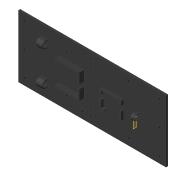
# Autodesk Inventor part: lowerBase
Saved by Autodesk Inventor 2019 (Build 230136000, 136)
## iProperties
Created: 2021-03-03
Part Number: lowerBase
Material: Generic
Document SubType Name: Modeling
Designer: LuoYi
Density: 1 g/cm^3
Appearance: Default
Author: LuoYi
Autodesk Inventor part; units mm, degrees
ref_plane "YZ Plane" through (0, 0, 0) normal (1, 0, 0) x (0, 1, 0)
ref_plane "XZ Plane" through (0, 0, 0) normal (0, 1, 0) x (-1, 0, 0)
ref_plane "XY Plane" through (0, 0, 0) normal (0, 0, 1) x (1, 0, 0)
sketch "Sketch1" plane through (0, 0, 0) normal (0, 0, 1) x (1, 0, 0)
  line L0 (0, 0) -> (200, 0)
  line L1 (200, 0) -> (200, 100)
  line L2 (200, 100) -> (0, 100)
  line L3 (0, 100) -> (0, 0)
  dimension "d0" = 200
  dimension "d1" = 100
  constraints: 8 end point, 2 parallel, 1 horizontal, 1 perpendicular
  measures "d0" distance of L2.end L1.end
  measures "d1" distance of L1.end L0.end
extrude "Extrusion1" add sketch "Sketch1" along normal blind 3
sketch "Sketch2" plane through (0, 0, 2) normal (-1, 0, 0) x (0, 0, 1)
  line L0 (1, 0) -> (1, 100) projected
  line L1 (1, 81.5) -> (5, 81.5)
  arc A0 (5, 73.5) -> (5, 81.5) centre (5, 77.5) ccw
  line L2 (5, 73.5) -> (1, 73.5)
  arc A1 (5, 71.5) -> (5, 83.5) centre (5, 77.5) ccw
  line L3 (5, 83.5) -> (1, 83.5)
  line L4 (5, 71.5) -> (1, 71.5)
  line L5 (1, 28.5) -> (5, 28.5)
  arc A2 (5, 16.5) -> (5, 28.5) centre (5, 22.5) ccw
  line L6 (5, 16.5) -> (1, 16.5)
  line L7 (1, 26.5) -> (5, 26.5)
  arc A3 (5, 18.5) -> (5, 26.5) centre (5, 22.5) ccw
  line L8 (5, 18.5) -> (1, 18.5)
  line L9 (1, 50) -> (8.8605, 50) construction
  line L10 (5, 77.5) -> (5, 22.5) construction
  point P0 (-2, 0)
  point P1 (5, 50)
  dimension "d4" = 8
  dimension "d5" = 2
  dimension "d6" = 2
  dimension "d7" = 8
  dimension "d8" = 55
  dimension "d9" = 4
  constraints: 20 end point, 9 horizontal, 8 point on circle, 8 tangent, 4 centre point, 2 coincident, 1 midpoint, 1 point on line, 1 vertical, 10 other
  measures "d4" distance between parallel lines of L8 L7
  measures "d5" distance between parallel lines of L5 L7
  measures "d6" distance between parallel lines of L2 L4
  measures "d7" distance between parallel lines of L2 L1
  measures "d8" distance of L10.start L10.end
extrude "Extrusion2" add sketch "Sketch2" against normal blind 10 contours L0 L2 A0 L1 L3 A1 L4 | L0 L8 A3 L7 L5 A2 L6
sketch "Sketch3" plane through (0, 0, 3) normal (0, 0, 1) x (1, 0, 0)
  line L0 (0, 71.5) -> (0, 28.5) projected
  line L1 (0, 50) -> (200, 50) construction
  line L2 (200, 0) -> (200, 100) projected
  line L3 (68, 30) -> (28, 30)
  line L4 (28, 30) -> (28, 70)
  line L5 (28, 70) -> (68, 70)
  line L6 (68, 70) -> (68, 30)
  line L7 (68, 30) -> (28, 70) construction
  line L8 (28, 30) -> (68, 70) construction
  line L9 (66, 32) -> (30, 32)
  line L10 (30, 32) -> (30, 68)
  line L11 (30, 68) -> (66, 68)
  line L12 (66, 68) -> (66, 32)
  line L13 (66, 32) -> (30, 68) construction
  line L14 (30, 32) -> (66, 68) construction
  line L15 (30, 68) -> (28, 68)
  line L16 (28, 68) -> (28, 32)
  line L17 (28, 32) -> (30, 32)
  line L18 (30, 32) -> (30, 68)
  line L19 (66, 46.75) -> (68, 46.75)
  line L20 (68, 46.75) -> (68, 53.25)
  line L21 (68, 53.25) -> (66, 53.25)
  line L22 (66, 53.25) -> (66, 46.75)
  point P0 (0, 0)
  point P1 (48, 50)
  point P2 (48, 50)
  point P3 (66, 50)
  dimension "d15" = 36
  dimension "d17" = 36
  dimension "d18" = 2
  dimension "d19" = 2
  dimension "d20" = 28
  dimension "d23" = 6.5
  constraints: 42 end point, 9 midpoint, 8 parallel, 4 horizontal, 4 perpendicular, 4 point on line, 1 collinear
  measures "d15" distance between parallel lines of L12 L10
  measures "d17" distance of L9.end L10.end
  measures "d18" distance between parallel lines of L5 L11
  measures "d19" distance between parallel lines of L4 L10
  measures "d20" distance between parallel lines of L0 L4
  measures "d23" distance between parallel lines of L21 L19
extrude "Extrusion3" add sketch "Sketch3" along normal blind 8 contours L3 L4 L17 L9 L12 L19 L6 | L21 L12 L11 L15 L4 L5 L6
sketch "Sketch4" plane through (0, 0, 3) normal (0, 0, 1) x (1, 0, 0)
  line L0 (0, 71.5) -> (0, 28.5) projected
  line L1 (200, 0) -> (200, 100) projected
  line L2 (100, 59) -> (130.2, 59)
  line L3 (130.2, 59) -> (130.2, 34.5)
  line L4 (130.2, 34.5) -> (100, 34.5)
  line L5 (100, 34.5) -> (100, 59)
  line L6 (98, 61) -> (132.2, 61)
  line L7 (132.2, 61) -> (132.2, 32.5)
  line L8 (132.2, 32.5) -> (98, 32.5)
  line L9 (98, 32.5) -> (98, 61)
  line L10 (88, 53.6) -> (98, 53.6) construction
  line L11 (98, 46.4) -> (88, 46.4) construction
  line L12 (88, 46.4) -> (88, 53.6) construction
  line L13 (88, 50) -> (0, 50) construction
  line L14 (68, 53.25) -> (68, 70) projected
  line L15 (98, 53.6) -> (100, 53.6)
  line L16 (98, 46.4) -> (100, 46.4)
  line L17 (130.2, 53.6) -> (132.2, 53.6)
  line L18 (130.2, 46.4) -> (132.2, 46.4)
  line L19 (105.149, 34.5) -> (105.149, 32.5)
  line L20 (129.3871, 34.5) -> (129.3871, 32.5)
  point P0 (0, 0)
  dimension "d24" = 24.5
  dimension "d25" = 30.2
  dimension "d26" = 2
  dimension "d27" = 2
  dimension "d28" = 2
  dimension "d29" = 2
  dimension "d30" = 7.2
  dimension "d31" = 10
  dimension "d32" = 20
  dimension "d33" = 9
  constraints: 36 end point, 16 point on line, 6 perpendicular, 5 parallel, 4 horizontal, 2 midpoint
  measures "d24" distance between parallel lines of L4 L2
  measures "d25" distance between parallel lines of L3 L5
  measures "d26" distance between parallel lines of L9 L5
  measures "d27" distance between parallel lines of L6 L2
  measures "d28" distance between parallel lines of L7 L3
  measures "d29" distance between parallel lines of L8 L4
  measures "d30" distance between parallel lines of L11 L10
  measures "d31" distance of L11.start L11.end
  measures "d32" distance between parallel lines of L14 L12
  measures "d33" distance between parallel lines of L2 L13
extrude "Extrusion4" add sketch "Sketch4" along normal blind 5 contours L5 L15 L9 L6 L7 L17 L3 L2 | L5 L4 L19 L8 L9 L16 | L18 L7 L8 L20 L4 L3
sketch "Sketch5" plane through (0, 0, 0) normal (-1, 0, 0) x (0, 0, 1)
  line L0 (0, 0) -> (0, 100) projected
  line L1 (3, 0) -> (3, 100) projected
  line L2 (0, 0) -> (3, 0)
  line L3 (3, 0) -> (3, 100)
  line L4 (3, 100) -> (0, 100)
  line L5 (0, 100) -> (0, 0)
  constraints: 8 end point, 2 parallel, 1 horizontal, 1 perpendicular
extrude "Extrusion5" add sketch "Sketch5" along normal blind 38
sketch "Sketch6" plane through (0, 0, 3) normal (0, 0, 1) x (1, 0, 0)
  circle A0 centre (-28, 10) radius 1.6
  circle A1 centre (140, 10) radius 1.6
  circle A2 centre (190, 10) radius 1.6
  circle A3 centre (190, 50) radius 1.6
  circle A4 centre (190, 90) radius 1.6
  circle A5 centre (140, 90) radius 1.6
  circle A6 centre (-28, 90) radius 1.6
  line L0 (-28, 90) -> (190, 90) construction
  line L1 (190, 90) -> (190, 10) construction
  line L2 (190, 10) -> (-28, 10) construction
  line L3 (-28, 10) -> (-28, 90) construction
  line L4 (200, 100) -> (-38, 100) projected
  line L5 (-38, 0) -> (-38, 100) projected
  line L6 (200, 0) -> (-38, 0) projected
  line L7 (200, 0) -> (200, 100) projected
  line L8 (-38, 50) -> (200, 50) construction
  circle A7 centre (-28, 50) radius 1.6
  line L9 (0, 83.5) -> (0, 71.5) projected
  line L10 (140, 90) -> (140, 10) construction
  line L11 (40, 80) -> (78.5, 80) construction
  line L12 (78.5, 80) -> (78.5, 20) construction
  line L13 (78.5, 20) -> (40, 20) construction
  line L14 (40, 20) -> (40, 80) construction
  circle A8 centre (40, 80) radius 1.6
  circle A9 centre (78.5, 80) radius 1.6
  circle A10 centre (40, 20) radius 1.6
  circle A11 centre (78.5, 20) radius 1.6
  point P0 (0, 0)
  dimension "d38" = 3.2
  dimension "d41" = 3.2
  dimension "d42" = 3.2
  dimension "d43" = 3.2
  dimension "d44" = 3.2
  dimension "d45" = 3.2
  dimension "d48" = 3.2
  dimension "d49" = 10
  dimension "d50" = 10
  dimension "d51" = 10
  dimension "d52" = 10
  dimension "d53" = 3.2
  dimension "d56" = 50
  dimension "d68" = 60
  dimension "d69" = 3.2
  dimension "d70" = 3.2
  dimension "d71" = 3.2
  dimension "d72" = 3.2
  dimension "d73" = 40
  dimension "d74" = 38.5
  constraints: 20 end point, 12 centre point, 4 coincident, 4 midpoint, 4 parallel, 3 point on line, 2 horizontal, 2 perpendicular, 1 vertical, 1 other
  measures "d38" diameter of A0
  measures "d41" diameter of A1
  measures "d42" diameter of A2
  measures "d43" diameter of A3
  measures "d44" diameter of A4
  measures "d45" diameter of A5
  measures "d48" diameter of A6
  measures "d49" distance between parallel lines of L4 L0
  measures "d50" distance between parallel lines of L5 L3
  measures "d51" distance between parallel lines of L6 L2
  measures "d52" distance between parallel lines of L7 L1
  measures "d53" diameter of A7
  measures "d56" distance of L10.start L0.end
  measures "d68" distance of L13.end L11.start
  measures "d69" diameter of A8
  measures "d70" diameter of A9
  measures "d71" diameter of A10
  measures "d72" diameter of A11
  measures "d73" distance between parallel lines of L9 L14
  measures "d74" distance of L11.start L11.end
extrude "Extrusion6" cut sketch "Sketch6" against normal blind 5 contours A0 | A1 | A2 | A3 | A4 | A5 | A6 | A7 | A8 | A9 | A10 | A11
ref_plane "Work Plane1" through (152.2, 32.5, 3) normal (1, 0, 0) x (0, 0, -1)
sketch "Sketch7" plane through (152.2, 32.5, 3) normal (1, 0, 0) x (0, 0, -1)
  line L0 (0, 13.9) -> (0, 2) projected
  line L1 (0, 13) -> (-5, 13)
  arc A0 (-5, 22) -> (-5, 13) centre (-5, 17.5) ccw
  line L2 (-5, 22) -> (0, 22)
  line L3 (0, 21.1) -> (0, 28.5) projected
  arc A1 (-5, 21) -> (-5, 14) centre (-5, 17.5) ccw
  line L4 (-5, 14) -> (0, 14)
  line L5 (-5, 21) -> (0, 21)
  line L6 (0, -32.5) -> (0, 67.5) projected
  line L7 (0, 13.9) -> (-5, 13.9) projected
  line L8 (0, 21.1) -> (-5, 21.1) projected
  line L9 (-5, 13.9) -> (-5, 21.1) construction
  line L10 (-5, 17.5) -> (-5, 17.5) construction
  point P0 (3, -32.5)
  point P1 (0, 0)
  dimension "d63" = 3.5
  dimension "d64" = 4.5
  dimension "d65" = 5
  constraints: 12 end point, 4 horizontal, 4 point on circle, 3 point on line, 2 centre point, 2 perpendicular, 1 coincident, 1 midpoint, 1 tangent, 2 other
  measures "d63" radius of A1
  measures "d64" radius of A0
  measures "d65" distance of L2.start L2.end
extrude "Extrusion7" add sketch "Sketch7" along normal blind 5 contours L0 L1 A0 L2 L3 L6 L5 A1 L4
sketch "Sketch9" plane through (0, 0, 3) normal (0, 0, 1) x (1, 0, 0)
  line L0 (65.5, 10) -> (78.5, 10) construction
  line L1 (78.5, 10) -> (78.5, 90) construction
  line L2 (78.5, 90) -> (65.5, 90) construction
  line L3 (65.5, 90) -> (65.5, 10) construction
  line L4 (65.5, 10) -> (78.5, 90) construction
  line L5 (78.5, 10) -> (65.5, 90) construction
  line L6 (-38, 100) -> (-38, 0) projected
  line L7 (-38, 50) -> (72, 50) construction
  circle A0 centre (65.5, 90) radius 1.6
  circle A1 centre (78.5, 90) radius 1.6
  circle A2 centre (65.5, 10) radius 1.6
  circle A3 centre (78.5, 10) radius 1.6
  circle A4 centre (-28, 90) radius 1.6 projected
  line L8 (-28, 90) -> (65.5, 90) construction
  point P0 (0, 0)
  dimension "d91" = 110
  dimension "d92" = 3.2
  dimension "d93" = 3.2
  dimension "d94" = 3.2
  dimension "d95" = 3.2
  dimension "d96" = 13
  constraints: 16 end point, 4 centre point, 4 coincident, 3 midpoint, 2 horizontal, 2 parallel, 2 perpendicular
  measures "d91" distance of L7.start L7.end
  measures "d92" diameter of A0
  measures "d93" diameter of A1
  measures "d94" diameter of A2
  measures "d95" diameter of A3
  measures "d96" distance of L1.end L2.end
extrude "Extrusion8" cut sketch "Sketch9" against normal blind 10 contours A0 | A1 | A2 | A3
equation "\"d50\" = d49"
equation "\"d51\" = d49"
equation "\"d52\" = d49"
body "Solid1"
